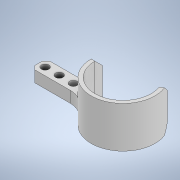
# Autodesk Inventor part: squirrely_leg
Saved by Autodesk Inventor 2020 (Build 240168000, 168)
## iProperties
Created: 2019-05-01
Part Number: squirrely_leg
Material: Generic
Document SubType Name: Modeling
Designer: mfans
Density: 1 g/cm^3
Appearance: Default
Author: mfans
Autodesk Inventor part; units mm, degrees
ref_plane "YZ Plane" through (0, 0, 0) normal (1, 0, 0) x (0, 1, 0)
ref_plane "XZ Plane" through (0, 0, 0) normal (0, 1, 0) x (-1, 0, 0)
ref_plane "XY Plane" through (0, 0, 0) normal (0, 0, 1) x (1, 0, 0)
sketch "Sketch1" plane through (0, 0, 0) normal (0, 1, 0) x (-1, 0, 0)
  line L0 (15, 4) -> (-15, 4)
  line L1 (-15, 4) -> (-15, -4)
  line L2 (-15, -4) -> (15, -4)
  line L3 (15, -4) -> (15, 4)
  line L4 (15, 4) -> (-15, -4) construction
  line L5 (-15, 4) -> (15, -4) construction
  point P0 (0, 0)
  dimension "d0" = 8
  dimension "d1" = 30
  constraints: 12 end point, 2 midpoint, 2 parallel, 1 horizontal, 1 perpendicular
  measures "d0" distance between parallel lines of L0 L2
  measures "d1" distance of L1.end L2.end
extrude "Extrusion1" add sketch "Sketch1" along normal blind 6
sketch "Sketch2" plane through (0, 6, 0) normal (0, 1, 0) x (1, 0, 0)
  line L0 (15, -4) -> (15, 4) projected
  line L1 (15, 4) -> (-15, 4) projected
  line L2 (-15, 4) -> (-15, -4) projected
  line L3 (-15, -4) -> (15, -4) projected
  point P0 (0, 0)
  point P1 (-4, 0)
  point P2 (-11.5, 0)
  point P3 (3.5, 0)
  dimension "d4" = 7.5
  dimension "d5" = 11
  dimension "d14" = 7.5
  measures "d4" distance of point (-11.5, 0) point (-4, 0)
  measures "d5" distance from line of L2 point (-4, 0)
  measures "d14" distance of point (-4, 0) point (3.5, 0)
hole "Hole1" at (-4, 6, 0) at (-11.5, 6, 0) at (3.5, 6, 0) direction (0, -1, 0) diameter 4 end through all
sketch "Sketch3" plane through (0, 6, 0) normal (0, 1, 0) x (1, 0, 0)
  line L0 (15, -4) -> (15, 4) projected
  arc A0 (15, 0) -> (42.1722, 8.7657) centre (30, 0) ccw
  arc A1 (13, 0) -> (43.912, 9.7702) centre (30, 0) ccw
  line L1 (43.912, 9.7702) -> (42.1722, 8.7657)
  line L2 (15, 0) -> (15, 4)
  line L3 (15, 4) -> (-15, 4) projected
  line L4 (13, 4) -> (13, 0)
  point P0 (0, 0)
  dimension "d15" = 2
  dimension "d16" = 0
  dimension "d17" = 60
  dimension "d22" = 15
  constraints: 6 end point, 4 point on circle, 3 tangent, 2 centre point, 1 coincident, 1 collinear, 1 midpoint, 1 point on line
  measures "d15" radial gap between concentric circles of A1 A0
  measures "d16" vertical distance of point (0, 0) A0.centre
  measures "d17" angle of L0 L1
  measures "d22" radius of A0
extrude "Extrusion2" add sketch "Sketch3" along normal blind 16 and the other way blind 6
chamfer "Chamfer1" distance 5 angle 45 2 edges at (13, 6, -2) (13.1197, 6, 2.0142)
chamfer "Chamfer2" distance 2 angle 45 2 edges at (-15, 3, 4) (-15, 3, -4)
chamfer "Chamfer3" distance 4 angle 45 3 edges at (14, 22, -4) (43.0421, 22, -9.2679) (43.0421, 0, -9.2679)
fillet "Fillet1" radius 12 2 edges at (13.4773, 8.5, 4) (13.4773, 3, 4)
fillet "Fillet2" radius 4 1 edges at (11.8549, 9.001, 5.6319)
body "Solid1"
